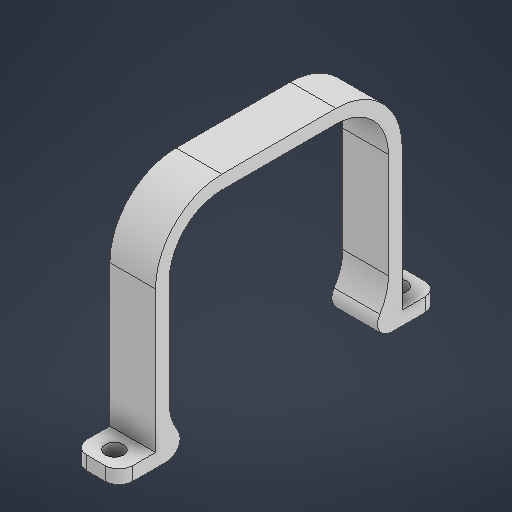
# Autodesk Inventor part: BatteryBracket
Saved by Autodesk Inventor 2026.1 (Build 301233000, 233)
## iProperties
Created: 2026-01-18
Part Number: BatteryBracket
Material: Generic
Document SubType Name: Modeling
Designer: Brynjar
Density: 1 g/cm^3
Appearance: Default
Author: Brynjar
Autodesk Inventor part; units mm, degrees
ref_plane "YZ Plane" through (0, 0, 0) normal (1, 0, 0) x (0, 1, 0)
ref_plane "XZ Plane" through (0, 0, 0) normal (0, 1, 0) x (-1, 0, 0)
ref_plane "XY Plane" through (0, 0, 0) normal (0, 0, 1) x (1, 0, 0)
derived "BatteryHolder.ipt"
sketch "Sketch1" plane through (0, 0, 0) normal (1, 0, 0) x (0, 1, 0)
  line L0 (-11.5, 20.5) -> (11.5, 20.5)
  line L1 (19.5, 12.5) -> (19.5, -12.5)
  line L2 (11.5, -20.5) -> (-11.5, -20.5)
  line L3 (-19.5, -12.5) -> (-19.5, 12.5)
  line L4 (-19.5, 20.5) -> (19.5, -20.5) construction
  line L5 (19.5, 20.5) -> (-19.5, -20.5) construction
  line L6 (-11.5, 23.5) -> (11.5, 23.5)
  line L7 (22.5, 12.5) -> (22.5, -12.5)
  line L8 (11.5, -23.5) -> (-11.5, -23.5)
  line L9 (-22.5, -12.5) -> (-22.5, 12.5)
  line L10 (-22.5, 23.5) -> (22.5, -23.5) construction
  line L11 (22.5, 23.5) -> (-22.5, -23.5) construction
  arc A0 (19.5, 12.5) -> (11.5, 20.5) centre (11.5, 12.5) ccw
  arc A1 (11.5, -20.5) -> (19.5, -12.5) centre (11.5, -12.5) ccw
  arc A2 (-19.5, -12.5) -> (-11.5, -20.5) centre (-11.5, -12.5) ccw
  arc A3 (-11.5, 20.5) -> (-19.5, 12.5) centre (-11.5, 12.5) ccw
  arc A4 (22.5, 12.5) -> (11.5, 23.5) centre (11.5, 12.5) ccw
  arc A5 (11.5, -23.5) -> (22.5, -12.5) centre (11.5, -12.5) ccw
  arc A6 (-22.5, -12.5) -> (-11.5, -23.5) centre (-11.5, -12.5) ccw
  arc A7 (-11.5, 23.5) -> (-22.5, 12.5) centre (-11.5, 12.5) ccw
  point P0 (0, 0)
sketch "Sketch2" plane through (0, 0, 0) normal (1, 0, 0) x (0, 1, 0)
  line L0 (22.5, 12.5) -> (22.5, -12.5) construction
  arc A0 (22.5, 12.5) -> (11.5, 23.5) centre (11.5, 12.5) ccw construction
  line L1 (-11.5, 23.5) -> (11.5, 23.5) construction
  arc A1 (-11.5, 23.5) -> (-22.5, 12.5) centre (-11.5, 12.5) ccw construction
  line L2 (-22.5, -12.5) -> (-22.5, 12.5) construction
  arc A2 (-22.5, -12.5) -> (-11.5, -23.5) centre (-11.5, -12.5) ccw construction
  line L3 (11.5, -23.5) -> (-11.5, -23.5) construction
  arc A3 (11.5, -23.5) -> (22.5, -12.5) centre (11.5, -12.5) ccw construction
  line L4 (23, -12.5) -> (23, 12.5)
  arc A4 (23, 12.5) -> (11.5, 24) centre (11.5, 12.5) ccw
  line L5 (11.5, 24) -> (-11.5, 24)
  arc A5 (-11.5, 24) -> (-23, 12.5) centre (-11.5, 12.5) ccw
  line L6 (-23, 12.5) -> (-23, -12.5) construction
  arc A6 (-23, -12.5) -> (-11.5, -24) centre (-11.5, -12.5) ccw
  line L7 (-11.5, -24) -> (11.5, -24)
  arc A7 (11.5, -24) -> (23, -12.5) centre (11.5, -12.5) ccw
  line L8 (26, 12.5) -> (26, -12.5)
  arc A8 (11.5, -27) -> (26, -12.5) centre (11.5, -12.5) ccw
  line L9 (11.5, -27) -> (-11.5, -27)
  arc A9 (-26, -12.5) -> (-11.5, -27) centre (-11.5, -12.5) ccw construction
  line L10 (-26, -12.5) -> (-26, 12.5) construction
  arc A10 (-11.5, 27) -> (-26, 12.5) centre (-11.5, 12.5) ccw construction
  line L11 (-11.5, 27) -> (11.5, 27)
  arc A11 (26, 12.5) -> (11.5, 27) centre (11.5, 12.5) ccw
  line L12 (-22.5, 12.5) -> (-22.5, 15.8541) construction
  line L13 (-22.5, 15.8541) -> (-22.5, 21.9472)
  line L14 (-22.5, 21.9472) -> (-22.5, 35)
  line L15 (-19.5, 24.5934) -> (-19.5, 27) construction
  line L16 (-11.5, 27) -> (-19.5, 27)
  line L17 (-19.5, 35) -> (-22.5, 35)
  line L18 (-19.5, 27) -> (-19.5, 35)
  line L19 (-22.5, 0) -> (22.5, 0) construction
  line L20 (-22.5, -15.8541) -> (-22.5, -21.9472)
  line L21 (-22.5, -21.9472) -> (-22.5, -35)
  line L22 (-11.5, -27) -> (-19.5, -27)
  line L23 (-19.5, -35) -> (-22.5, -35)
  line L24 (-19.5, -27) -> (-19.5, -35)
  point P0 (0, 0)
  dimension "d1" = 0.5
  dimension "d2" = 3
  dimension "d3" = 3
  dimension "d4" = 8
  constraints: 42 end point, 19 point on circle, 8 centre point, 5 symmetric about line, 4 point on line, 2 midpoint, 2 perpendicular, 2 vertical, 1 horizontal, 14 other
  measures "d1" distance between parallel lines of L0 L4
  measures "d2" distance between parallel lines of L4 L8
  measures "d3" distance of L17.start L14.end
  measures "d4" distance of L15.end L17.start
extrude "Extrusion1" add sketch "Sketch2" along normal blind 10
fillet "Fillet1" radius 3 6 edges at (5, -22.5, -15.8541) (5, -22.5, 15.8541) (10, -21, -35) (0, -21, -35) (10, -21, 35) (0, -21, 35)
sketch "Sketch3" plane through (0, -19.5, 27) normal (0, 1, 0) x (1, 0, 0)
  circle A0 centre (5, -4) radius 2
  circle A1 centre (5, 58) radius 2
  line L0 (3, -8) -> (7, -8) construction
  line L1 (5, -8) -> (5, -4) construction
  line L2 (0, 0) -> (10, 0) construction
  line L3 (5, 0) -> (5, -4) construction
  line L4 (0, 27) -> (10, 27) construction
  line L5 (10, 14.5) -> (10, 39.5) construction
  dimension "d8" = 4
  constraints: 6 end point, 3 midpoint, 2 centre point, 1 collinear, 1 equal radius, 1 perpendicular, 1 vertical, 1 other
  measures "d8" diameter of A0
extrude "Extrusion2" cut sketch "Sketch3" against normal through all
body "Solid1"
